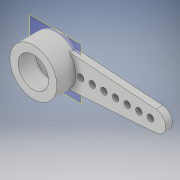
# Autodesk Inventor part: singleSideCutoff
Saved by Autodesk Inventor 2017 (Build 210142000, 142)
## iProperties
Created: 2016-12-06
Part Number: singleSideCutoff
Material: Generic
Document SubType Name: Modeling
Designer: PLTW
Density: 1 g/cm^3
Appearance: Default
Author: PLTW
Autodesk Inventor part; units mm, degrees
ref_plane "YZ Plane" through (0, 0, 0) normal (1, 0, 0) x (0, 1, 0)
ref_plane "XZ Plane" through (0, 0, 0) normal (0, 1, 0) x (-1, 0, 0)
ref_plane "XY Plane" through (0, 0, 0) normal (0, 0, 1) x (1, 0, 0)
sketch "Sketch1" plane through (0, 0, 0) normal (0, 0, 1) x (1, 0, 0)
  circle A0 centre (0, 0) radius 3.6957
  dimension "d0" = 7.3914
  constraints: 1 centre point, 1 coincident
  measures "d0" diameter of A0
extrude "Extrusion1" add sketch "Sketch1" along normal blind 4.0386
sketch "Sketch2" plane through (0, 0, 4.0386) normal (0, 0, 1) x (1, 0, 0)
  circle A0 centre (0, 0) radius 3.6957 projected
  circle A1 centre (0, 0) radius 2.4003
  dimension "d3" = 1.2954
  constraints: 1 centre point, 1 coincident
  measures "d3" radial gap between concentric circles of A1 A0
extrude "Extrusion2" cut sketch "Sketch2" against normal blind 2.7432 contours A1
sketch "Sketch3" plane through (0, 0, 0) normal (0, 0, -1) x (-1, 0, 0)
  circle A0 centre (0, 0) radius 3.6957 projected
  circle A1 centre (0, 0) radius 2.1717
  dimension "d6" = 1.524
  constraints: 1 centre point, 1 coincident
  measures "d6" radial gap between concentric circles of A1 A0
extrude "Extrusion3" cut sketch "Sketch3" against normal blind 1.0668 contours A1
sketch "Sketch4" plane through (0, 0, 1.2954) normal (0, 0, 1) x (1, 0, 0)
  circle A0 centre (0, 0) radius 2.4003 projected
  circle A1 centre (0, 0) radius 1.4478
  dimension "d9" = 2.8956
  constraints: 1 centre point, 1 coincident
  measures "d9" diameter of A1
extrude "Extrusion4" cut sketch "Sketch4" against normal through all contours A1
ref_plane "Work Plane1" through (0, 0, 0.5334) normal (0, 0, -1) x (-1, 0, 0)
sketch "Sketch5" plane through (0, 0, 0.5334) normal (0, 0, -1) x (-1, 0, 0)
  circle A0 centre (0, 0) radius 3.6957 projected
  line L0 (-2.6602, 2.5654) -> (-16.3171, 1.6256)
  line L1 (-2.6602, -2.5654) -> (-16.3171, -1.6256)
  arc A1 (-16.3171, 1.6256) -> (-16.3171, -1.6256) centre (-16.2052, 0) ccw
  circle A2 centre (0, 0) radius 2.4003 projected
  line L2 (2.6602, 2.5654) -> (16.3171, 1.6256)
  arc A3 (16.3171, -1.6256) -> (16.3171, 1.6256) centre (16.2052, 0) ccw
  line L3 (2.6602, -2.5654) -> (16.3171, -1.6256)
  dimension "d12" = 5.1308
  dimension "d15" = 16.2052
  dimension "d28" = 360
  dimension "d35" = 3.2512
  constraints: 8 end point, 6 point on circle, 2 centre point, 2 tangent, 1 equal length, 1 horizontal alignment, 17 other
  measures "d12" distance of L1.start L0.start
  measures "d15" distance of A1.centre point (0, 0)
  measures "d35" distance of L1.end L0.end
extrude "Extrusion5" add sketch "Sketch5" along normal mid plane 1.0668 contours A0 L1 A1 L0
sketch "Sketch6" plane through (0, 0, 0) normal (0, 0, -1) x (-1, 0, 0)
  circle A0 centre (0, 0) radius 2.1717 projected
  circle A1 centre (-4.4831, 0) radius 0.508
  dimension "d36" = 1.8034
  dimension "d37" = 1.016
  constraints: 1 centre point, 1 horizontal alignment
  measures "d37" diameter of A1
extrude "Extrusion6" cut sketch "Sketch6" against normal through all contours A1
pattern_linear "Rectangular Pattern1" count 7 spacing 1.8288 along (1, 0, 0) of "Extrusion6"
body "Solid1"
